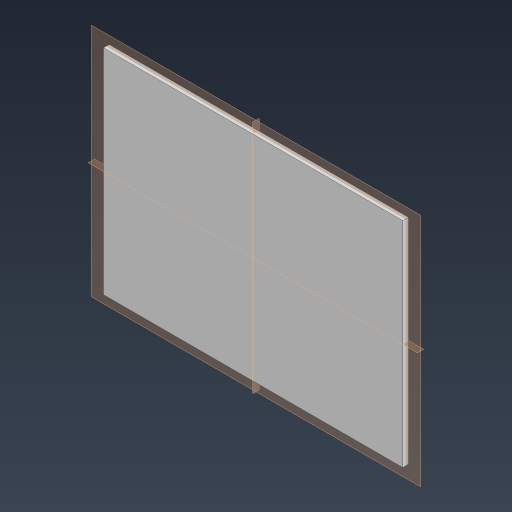
# Autodesk Inventor part: Панель_крепления_моторов
Saved by Autodesk Inventor 2023.2 (Build 272271030, 271C)
## iProperties
Created: 2025-12-09
Part Number: Панель_крепления_моторов
Material: Типовые
Document SubType Name: Modeling
Designer: Олег Коноваленко
Density: 1 g/cm^3
Appearance: По умолчанию
Author: Олег Коноваленко
Autodesk Inventor part; units mm, degrees
sketch "Эскиз1" plane through (0, 0, 0) normal (0, 0, 1) x (1, 0, 0)
  line L0 (-105, -75) -> (105, -75)
  line L1 (105, -75) -> (105, 75)
  line L2 (105, 75) -> (-105, 75)
  line L3 (-105, 75) -> (-105, -75)
  line L4 (-105, -75) -> (105, 75) construction
  line L5 (105, -75) -> (-105, 75) construction
  point P0 (0, 0)
  dimension "d0" = 210
  dimension "d1" = 150
  constraints: 12 end point, 2 midpoint, 2 parallel, 1 horizontal, 1 perpendicular
  measures "d0" distance of L1.end L2.end
  measures "d1" distance of L2.end L0.start
extrude "Выдавливание1" add sketch "Эскиз1" along normal mid plane 4
